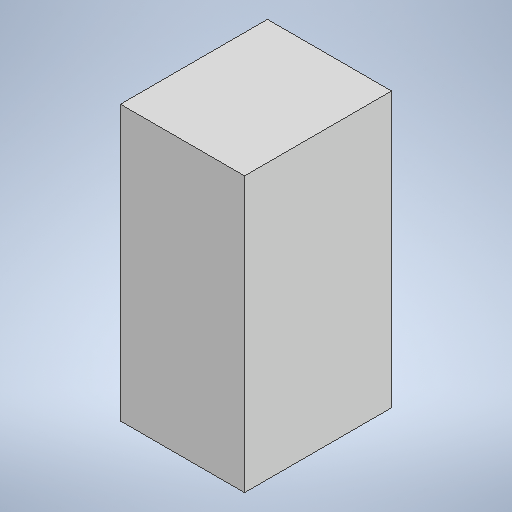
# Autodesk Inventor part: Air Conditioning Unit
Saved by Autodesk Inventor 2025 (Build 290162010, 162A)
## iProperties
Created: 2024-06-12
Part Number: Air Conditioning Unit
Material: Generic
Document SubType Name: Modeling
Designer: Alan Thomas
Mass: 143640 g
Surface Area: 17364 cm^2
Volume: 143640 cm^3
Density: 1 g/cm^3
Appearance: Default
Author: Alan Thomas
Autodesk Inventor part; units mm, degrees
ref_plane "YZ Plane" through (0, 0, 0) normal (1, 0, 0) x (0, 1, 0)
ref_plane "XZ Plane" through (0, 0, 0) normal (0, 1, 0) x (-1, 0, 0)
ref_plane "XY Plane" through (0, 0, 0) normal (0, 0, 1) x (1, 0, 0)
sketch "Sketch1" plane through (0, 0, 0) normal (0, 1, 0) x (-1, 0, 0)
  line L0 (0, 0) -> (12.8026, 0)
  line L1 (0, 0) -> (380, 0)
  line L2 (380, 0) -> (380, -450)
  line L3 (380, -450) -> (0, -450)
  line L4 (0, -450) -> (0, 0)
  dimension "d0" = 380
  dimension "d1" = 450
  constraints: 10 end point, 2 horizontal, 2 parallel, 1 perpendicular
  measures "d0" distance of L2.end L3.end
  measures "d1" distance of L1.end L2.end
extrude "Extrusion1" add sketch "Sketch1" along normal blind 840
body "Solid1"
